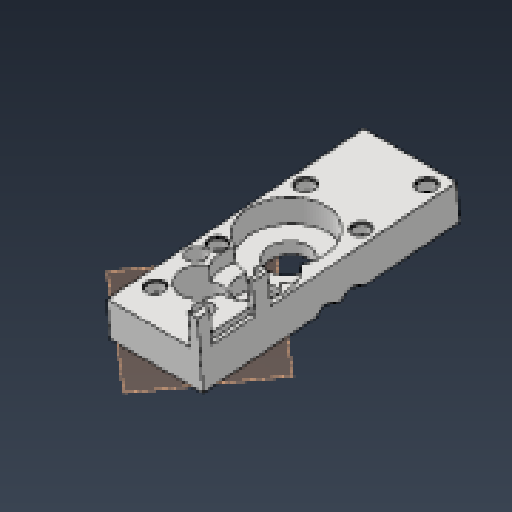
# Autodesk Inventor part: Right_gearbox
Saved by Autodesk Inventor 2026.2 (Build 302298010, 298A)
## iProperties
Created: 2026-04-04
Part Number: Right_gearbox
Material: Generic
Document SubType Name: Modeling
Designer: szymo
Density: 1 g/cm^3
Appearance: Default
Mass: 7.93657 g
Surface Area: 65.2995 cm^2
Volume: 7.93657 cm^3
Author: szymo
Autodesk Inventor part; units mm, degrees
(part 1 of 2)
ref_plane "YZ Plane" through (0, 0, 0) normal (1, 0, 0) x (0, 1, 0)
ref_plane "XZ Plane" through (0, 0, 0) normal (0, 1, 0) x (-1, 0, 0)
ref_plane "XY Plane" through (0, 0, 0) normal (0, 0, 1) x (1, 0, 0)
ref_plane "Work Plane1" through (-23.7091, -17.2437, 13.99) normal (0, 0.9970894, 0.0762418) x (-1, 0, 0)
sketch "Sketch1" plane through (-23.7091, -17.2437, 13.99) normal (0, 0.9970894, 0.0762418) x (-1, 0, 0)
  line L0 (-0.0409, -0.625) -> (23.5591, -0.625)
  line L1 (23.5591, -0.625) -> (23.5591, -65.9208)
  line L2 (23.5591, -65.9208) -> (-0.0409, -65.9208)
  line L3 (-0.0409, -65.9208) -> (-0.0409, -0.625)
  circle A0 centre (9.1675, -23.6102) radius 8 construction
  circle A1 centre (12.9591, -35.6262) radius 9.6 construction
  circle A2 centre (9.1675, -23.6102) radius 8.4
  circle A3 centre (12.9591, -35.6262) radius 10
  circle A4 centre (9.1675, -23.6102) radius 4.2 construction
  circle A5 centre (9.1675, -23.6102) radius 4.6
  line L4 (20.6624, -53.9792) -> (25.4482, -49.9634)
  arc A6 (25.4482, -49.9634) -> (22.2343, -46.1332) centre (14.4591, -55.9208) ccw
  line L5 (22.2343, -46.1332) -> (17.4484, -50.149)
  arc A7 (20.6624, -53.9792) -> (17.4484, -50.149) centre (14.4591, -55.9208) ccw
  arc A8 (3.4701, -61.8782) -> (6.684, -65.7084) centre (14.4591, -55.9208) ccw
  line L6 (3.4701, -61.8782) -> (8.2559, -57.8624)
  arc A9 (8.2559, -57.8624) -> (11.4698, -61.6927) centre (14.4591, -55.9208) ccw
  line L7 (11.4698, -61.6927) -> (6.684, -65.7084)
  line L8 (6.684, -65.7084) -> (6.684, -65.9208)
  line L9 (11.4698, -61.6927) -> (23.5591, -61.6927)
  circle A10 centre (14.4591, -15.125) radius 5 projected
  circle A11 centre (14.4591, -15.125) radius 13.85 construction
  circle A12 centre (14.4591, -55.9208) radius 14.5 construction
  circle A13 centre (14.4591, -15.125) radius 14.5 construction
  line L10 (19.1242, -50.0482) -> (22.2292, -47.4428) construction
  arc A14 (24.1576, -49.741) -> (22.2292, -47.4428) centre (14.4591, -55.9208) ccw construction
  line L11 (24.1576, -49.741) -> (21.0526, -52.3464) construction
  arc A15 (21.0526, -52.3464) -> (19.1242, -50.0482) centre (14.4591, -55.9208) ccw construction
  arc A16 (4.7607, -62.1007) -> (6.6891, -64.3988) centre (14.4591, -55.9208) ccw construction
  line L12 (4.7607, -62.1007) -> (7.8657, -59.4953) construction
  arc A17 (7.8657, -59.4953) -> (9.7941, -61.7934) centre (14.4591, -55.9208) ccw construction
  line L13 (9.7941, -61.7934) -> (6.6891, -64.3988) construction
  circle A18 centre (14.4591, -55.9208) radius 5 projected
  circle A19 centre (14.4591, -55.9208) radius 13.85 projected
  circle A20 centre (12.9591, -35.6262) radius 5 projected
  circle A21 centre (9.1675, -23.6102) radius 1.25 projected
  arc A22 (5.3654, -25.3945) -> (6.7676, -25.1474) centre (5.4355, -21.6906) ccw projected
  arc A23 (6.7676, -25.1474) -> (6.9888, -25.4475) centre (9.1675, -23.6102) ccw projected
  arc A24 (6.9888, -25.4475) -> (6.3377, -26.7137) centre (9.8963, -27.7432) ccw projected
  arc A25 (6.3377, -26.7137) -> (6.767, -27.0565) centre (9.1675, -23.6102) ccw projected
  arc A26 (6.767, -27.0565) -> (7.8577, -26.1414) centre (4.9757, -23.8138) ccw projected
  arc A27 (7.8577, -26.1414) -> (8.1993, -26.2907) centre (9.1675, -23.6102) ccw projected
  arc A28 (8.1993, -26.2907) -> (8.2685, -27.7129) centre (11.8651, -26.8251) ccw projected
  arc A29 (8.2685, -27.7129) -> (8.8117, -27.7951) centre (9.1675, -23.6102) ccw projected
  arc A30 (8.8117, -27.7951) -> (9.2988, -26.4572) centre (5.6391, -25.8824) ccw projected
  arc A31 (9.2988, -26.4572) -> (9.6693, -26.4157) centre (9.1675, -23.6102) ccw projected
  arc A32 (9.6693, -26.4157) -> (10.4403, -27.6127) centre (13.1112, -25.0456) ccw projected
  arc A33 (10.4403, -27.6127) -> (10.9519, -27.4123) centre (9.1675, -23.6102) ccw projected
  arc A34 (10.9519, -27.4123) -> (10.7047, -26.0101) centre (7.248, -27.3422) ccw projected
  arc A35 (10.7047, -26.0101) -> (11.0048, -25.7889) centre (9.1675, -23.6102) ccw projected
  arc A36 (11.0048, -25.7889) -> (12.271, -26.4401) centre (13.3005, -22.8814) ccw projected
  arc A37 (12.271, -26.4401) -> (12.6139, -26.0108) centre (9.1675, -23.6102) ccw projected
  arc A38 (12.6139, -26.0108) -> (11.6987, -24.92) centre (9.3712, -27.802) ccw projected
  arc A39 (11.6987, -24.92) -> (11.848, -24.5784) centre (9.1675, -23.6102) ccw projected
  arc A40 (11.848, -24.5784) -> (13.2702, -24.5092) centre (12.3824, -20.9126) ccw projected
  arc A41 (13.2702, -24.5092) -> (13.3524, -23.966) centre (9.1675, -23.6102) ccw projected
  arc A42 (13.3524, -23.966) -> (12.0145, -23.4789) centre (11.4398, -27.1386) ccw projected
  arc A43 (12.0145, -23.4789) -> (11.973, -23.1084) centre (9.1675, -23.6102) ccw projected
  arc A44 (11.973, -23.1084) -> (13.17, -22.3374) centre (10.6029, -19.6665) ccw projected
  arc A45 (13.17, -22.3374) -> (12.9697, -21.8259) centre (9.1675, -23.6102) ccw projected
  arc A46 (12.9697, -21.8259) -> (11.5674, -22.073) centre (12.8996, -25.5298) ccw projected
  arc A47 (11.5674, -22.073) -> (11.3463, -21.7729) centre (9.1675, -23.6102) ccw projected
  arc A48 (11.3463, -21.7729) -> (11.9974, -20.5067) centre (8.4388, -19.4772) ccw projected
  arc A49 (11.9974, -20.5067) -> (11.5681, -20.1639) centre (9.1675, -23.6102) ccw projected
  arc A50 (11.5681, -20.1639) -> (10.4773, -21.079) centre (13.3593, -23.4066) ccw projected
  arc A51 (10.4773, -21.079) -> (10.1357, -20.9297) centre (9.1675, -23.6102) ccw projected
  arc A52 (10.1357, -20.9297) -> (10.0665, -19.5075) centre (6.4699, -20.3953) ccw projected
  arc A53 (10.0665, -19.5075) -> (9.5233, -19.4253) centre (9.1675, -23.6102) ccw projected
  arc A54 (9.5233, -19.4253) -> (9.0362, -20.7632) centre (12.6959, -21.3379) ccw projected
  arc A55 (9.0362, -20.7632) -> (8.6657, -20.8047) centre (9.1675, -23.6102) ccw projected
  arc A56 (8.6657, -20.8047) -> (7.8947, -19.6077) centre (5.2239, -22.1748) ccw projected
  arc A57 (7.8947, -19.6077) -> (7.3832, -19.8081) centre (9.1675, -23.6102) ccw projected
  arc A58 (7.3832, -19.8081) -> (7.6303, -21.2103) centre (11.0871, -19.8782) ccw projected
  arc A59 (7.6303, -21.2103) -> (7.3302, -21.4315) centre (9.1675, -23.6102) ccw projected
  arc A60 (7.3302, -21.4315) -> (6.064, -20.7803) centre (5.0345, -24.339) ccw projected
  arc A61 (6.064, -20.7803) -> (5.7212, -21.2096) centre (9.1675, -23.6102) ccw projected
  arc A62 (5.7212, -21.2096) -> (6.6363, -22.3004) centre (8.9639, -19.4184) ccw projected
  arc A63 (6.6363, -22.3004) -> (6.487, -22.642) centre (9.1675, -23.6102) ccw projected
  arc A64 (6.487, -22.642) -> (5.0649, -22.7112) centre (5.9526, -26.3078) ccw projected
  arc A65 (5.0649, -22.7112) -> (4.9826, -23.2544) centre (9.1675, -23.6102) ccw projected
  arc A66 (4.9826, -23.2544) -> (6.3206, -23.7415) centre (6.8953, -20.0818) ccw projected
  arc A67 (6.3206, -23.7415) -> (6.362, -24.112) centre (9.1675, -23.6102) ccw projected
  arc A68 (6.362, -24.112) -> (5.165, -24.883) centre (7.7322, -27.5539) ccw projected
  arc A69 (5.165, -24.883) -> (5.3654, -25.3945) centre (9.1675, -23.6102) ccw projected
  circle A70 centre (9.1675, -23.6102) radius 1.25 projected
  arc A71 (17.1384, -22.9282) -> (15.9774, -22.6664) centre (15.4653, -27.6426) ccw projected
  arc A72 (15.9774, -22.6664) -> (15.9187, -22.3113) centre (9.1675, -23.6102) ccw projected
  arc A73 (15.9187, -22.3113) -> (16.9336, -21.6897) centre (13.8318, -17.7649) ccw projected
  arc A74 (16.9336, -21.6897) -> (16.8224, -21.2858) centre (9.1675, -23.6102) ccw projected
  arc A75 (16.8224, -21.2858) -> (15.6324, -21.2712) centre (16.1661, -26.2451) ccw projected
  arc A76 (15.6324, -21.2712) -> (15.5011, -20.936) centre (9.1675, -23.6102) ccw projected
  arc A77 (15.5011, -20.936) -> (16.3646, -20.117) centre (12.5145, -16.9228) ccw projected
  arc A78 (16.3646, -20.117) -> (16.1719, -19.7451) centre (9.1675, -23.6102) ccw projected
  arc A79 (16.1719, -19.7451) -> (15.0048, -19.9781) centre (16.561, -24.7325) ccw projected
  arc A80 (15.0048, -19.9781) -> (14.8067, -19.6776) centre (9.1675, -23.6102) ccw projected
  arc A81 (14.8067, -19.6776) -> (15.481, -18.697) centre (11.051, -16.3731) ccw projected
  arc A82 (15.481, -18.697) -> (15.2152, -18.3733) centre (9.1675, -23.6102) ccw projected
  arc A83 (15.2152, -18.3733) -> (14.1221, -18.8439) centre (16.6328, -23.1708) ccw projected
  arc A84 (14.1221, -18.8439) -> (13.8659, -18.5911) centre (9.1675, -23.6102) ccw projected
  arc A85 (13.8659, -18.5911) -> (14.3215, -17.4917) centre (9.5052, -16.1397) ccw projected
  arc A86 (14.3215, -17.4917) -> (13.9942, -17.2303) centre (9.1675, -23.6102) ccw projected
  arc A87 (13.9942, -17.2303) -> (13.0229, -17.9179) centre (16.3783, -21.6283) ccw projected
  arc A88 (13.0229, -17.9179) -> (12.7197, -17.7239) centre (9.1675, -23.6102) ccw projected
  arc A89 (12.7197, -17.7239) -> (12.9368, -16.5538) centre (7.9446, -16.2327) ccw projected
  arc A90 (12.9368, -16.5538) -> (12.5623, -16.3662) centre (9.1675, -23.6102) ccw projected
  arc A91 (12.5623, -16.3662) -> (11.7551, -17.2407) centre (15.8086, -20.1724) ccw projected
  arc A92 (11.7551, -17.2407) -> (11.4182, -17.114) centre (9.1675, -23.6102) ccw projected
  arc A93 (11.4182, -17.114) -> (11.3873, -15.9243) centre (6.4374, -16.6482) ccw projected
  arc A94 (11.3873, -15.9243) -> (10.982, -15.8187) centre (9.1675, -23.6102) ccw projected
  arc A95 (10.982, -15.8187) -> (10.3743, -16.8419) centre (14.9487, -18.8667) ccw projected
  arc A96 (10.3743, -16.8419) -> (10.0184, -16.7881) centre (9.1675, -23.6102) ccw projected
  arc A97 (10.0184, -16.7881) -> (9.7408, -15.6308) centre (5.0496, -17.3679) ccw projected
  arc A98 (9.7408, -15.6308) -> (9.3224, -15.6117) centre (9.1675, -23.6102) ccw projected
  arc A99 (9.3224, -15.6117) -> (8.9407, -16.7389) centre (13.8362, -17.7684) ccw projected
  arc A100 (8.9407, -16.7389) -> (8.5814, -16.7602) centre (9.1675, -23.6102) ccw projected
  arc A101 (8.5814, -16.7602) -> (8.0693, -15.6859) centre (3.8418, -18.3605) ccw projected
  arc A102 (8.0693, -15.6859) -> (7.6561, -15.7543) centre (9.1675, -23.6102) ccw projected
  arc A103 (7.6561, -15.7543) -> (7.5171, -16.9362) centre (12.5196, -16.9254) ccw projected
  arc A104 (7.5171, -16.9362) -> (7.17, -17.0318) centre (9.1675, -23.6102) ccw projected
  arc A105 (7.17, -17.0318) -> (6.4457, -16.0874) centre (2.8667, -19.5825) ccw projected
  arc A106 (6.4457, -16.0874) -> (6.0558, -16.2402) centre (9.1675, -23.6102) ccw projected
  arc A107 (6.0558, -16.2402) -> (6.1655, -17.4252) centre (11.0565, -16.3745) ccw projected
  arc A108 (6.1655, -17.4252) -> (5.846, -17.5908) centre (9.1675, -23.6102) ccw projected
  arc A109 (5.846, -17.5908) -> (4.9411, -16.8177) centre (2.167, -20.9806) ccw projected
  arc A110 (4.9411, -16.8177) -> (4.5914, -17.0482) centre (9.1675, -23.6102) ccw projected
  arc A111 (4.5914, -17.0482) -> (4.9452, -18.1845) centre (9.5108, -16.1399) ccw projected
  arc A112 (4.9452, -18.1845) -> (4.667, -18.413) centre (9.1675, -23.6102) ccw projected
  arc A113 (4.667, -18.413) -> (3.6213, -17.8449) centre (1.7732, -22.4935) ccw projected
  arc A114 (3.6213, -17.8449) -> (3.3271, -18.143) centre (9.1675, -23.6102) ccw projected
  arc A115 (3.3271, -18.143) -> (3.9094, -19.181) centre (7.9502, -16.2318) ccw projected
  arc A116 (3.9094, -19.181) -> (3.6848, -19.4622) centre (9.1675, -23.6102) ccw projected
  arc A117 (3.6848, -19.4622) -> (2.5438, -19.124) centre (1.7026, -24.0553) ccw projected
  arc A118 (2.5438, -19.124) -> (2.3181, -19.4768) centre (9.1675, -23.6102) ccw projected
  arc A119 (2.3181, -19.4768) -> (3.1034, -20.371) centre (6.4427, -16.6461) ccw projected
  arc A120 (3.1034, -20.371) -> (2.9422, -20.6928) centre (9.1675, -23.6102) ccw projected
  arc A121 (2.9422, -20.6928) -> (1.7558, -20.5992) centre (1.9583, -25.5976) ccw projected
  arc A122 (1.7558, -20.5992) -> (1.6084, -20.9912) centre (9.1675, -23.6102) ccw projected
  arc A123 (1.6084, -20.9912) -> (2.5625, -21.7026) centre (5.0543, -17.3648) ccw projected
  arc A124 (2.5625, -21.7026) -> (2.4717, -22.0509) centre (9.1675, -23.6102) ccw projected
  arc A125 (2.4717, -22.0509) -> (1.2917, -22.206) centre (2.529, -27.0531) ccw projected
  arc A126 (1.2917, -22.206) -> (1.229, -22.6201) centre (9.1675, -23.6102) ccw projected
  arc A127 (1.229, -22.6201) -> (2.3102, -23.1175) centre (3.8457, -18.3565) ccw projected
  arc A128 (2.3102, -23.1175) -> (2.2938, -23.4771) centre (9.1675, -23.6102) ccw projected
  arc A129 (2.2938, -23.4771) -> (1.1719, -23.8741) centre (3.3899, -28.3581) ccw projected
  arc A130 (1.1719, -23.8741) -> (1.1967, -24.2922) centre (9.1675, -23.6102) ccw projected
  arc A131 (1.1967, -24.2922) -> (2.3576, -24.554) centre (2.8697, -19.5777) ccw projected
  arc A132 (2.3576, -24.554) -> (2.4163, -24.9091) centre (9.1675, -23.6102) ccw projected
  arc A133 (2.4163, -24.9091) -> (1.4015, -25.5307) centre (4.5033, -29.4555) ccw projected
  arc A134 (1.4015, -25.5307) -> (1.5126, -25.9345) centre (9.1675, -23.6102) ccw projected
  arc A135 (1.5126, -25.9345) -> (2.7027, -25.9492) centre (2.169, -20.9752) ccw projected
  arc A136 (2.7027, -25.9492) -> (2.8339, -26.2844) centre (9.1675, -23.6102) ccw projected
  arc A137 (2.8339, -26.2844) -> (1.9705, -27.1034) centre (5.8205, -30.2975) ccw projected
  arc A138 (1.9705, -27.1034) -> (2.1632, -27.4753) centre (9.1675, -23.6102) ccw projected
  arc A139 (2.1632, -27.4753) -> (3.3302, -27.2422) centre (1.7741, -22.4879) ccw projected
  arc A140 (3.3302, -27.2422) -> (3.5283, -27.5428) centre (9.1675, -23.6102) ccw projected
  arc A141 (3.5283, -27.5428) -> (2.854, -28.5234) centre (7.2841, -30.8473) ccw projected
  arc A142 (2.854, -28.5234) -> (3.1198, -28.8471) centre (9.1675, -23.6102) ccw projected
  arc A143 (3.1198, -28.8471) -> (4.213, -28.3765) centre (1.7023, -24.0496) ccw projected
  arc A144 (4.213, -28.3765) -> (4.4692, -28.6293) centre (9.1675, -23.6102) ccw projected
  arc A145 (4.4692, -28.6293) -> (4.0135, -29.7287) centre (8.8299, -31.0807) ccw projected
  arc A146 (4.0135, -29.7287) -> (4.3408, -29.9901) centre (9.1675, -23.6102) ccw projected
  arc A147 (4.3408, -29.9901) -> (5.3122, -29.3025) centre (1.9568, -25.5921) ccw projected
  arc A148 (5.3122, -29.3025) -> (5.6154, -29.4964) centre (9.1675, -23.6102) ccw projected
  arc A149 (5.6154, -29.4964) -> (5.3983, -30.6666) centre (10.3905, -30.9877) ccw projected
  arc A150 (5.3983, -30.6666) -> (5.7727, -30.8542) centre (9.1675, -23.6102) ccw projected
  arc A151 (5.7727, -30.8542) -> (6.5799, -29.9797) centre (2.5264, -27.048) ccw projected
  arc A152 (6.5799, -29.9797) -> (6.9168, -30.1063) centre (9.1675, -23.6102) ccw projected
  arc A153 (6.9168, -30.1063) -> (6.9477, -31.2961) centre (11.8976, -30.5722) ccw projected
  arc A154 (6.9477, -31.2961) -> (7.353, -31.4017) centre (9.1675, -23.6102) ccw projected
  arc A155 (7.353, -31.4017) -> (7.9608, -30.3785) centre (3.3863, -28.3537) ccw projected
  arc A156 (7.9608, -30.3785) -> (8.3166, -30.4323) centre (9.1675, -23.6102) ccw projected
  arc A157 (8.3166, -30.4323) -> (8.5942, -31.5896) centre (13.2855, -29.8524) ccw projected
  arc A158 (8.5942, -31.5896) -> (9.0126, -31.6087) centre (9.1675, -23.6102) ccw projected
  arc A159 (9.0126, -31.6087) -> (9.3943, -30.4815) centre (4.4989, -29.452) ccw projected
  arc A160 (9.3943, -30.4815) -> (9.7536, -30.4602) centre (9.1675, -23.6102) ccw projected
  arc A161 (9.7536, -30.4602) -> (10.2658, -31.5345) centre (14.4933, -28.8599) ccw projected
  arc A162 (10.2658, -31.5345) -> (10.679, -31.4661) centre (9.1675, -23.6102) ccw projected
  arc A163 (10.679, -31.4661) -> (10.818, -30.2841) centre (5.8155, -30.295) ccw projected
  arc A164 (10.818, -30.2841) -> (11.165, -30.1886) centre (9.1675, -23.6102) ccw projected
  arc A165 (11.165, -30.1886) -> (11.8893, -31.1329) centre (15.4684, -27.6379) ccw projected
  arc A166 (11.8893, -31.1329) -> (12.2793, -30.9802) centre (9.1675, -23.6102) ccw projected
  arc A167 (12.2793, -30.9802) -> (12.1695, -29.7952) centre (7.2786, -30.8459) ccw projected
  arc A168 (12.1695, -29.7952) -> (12.4891, -29.6296) centre (9.1675, -23.6102) ccw projected
  arc A169 (12.4891, -29.6296) -> (13.3939, -30.4027) centre (16.1681, -26.2398) ccw projected
  arc A170 (13.3939, -30.4027) -> (13.7436, -30.1722) centre (9.1675, -23.6102) ccw projected
  arc A171 (13.7436, -30.1722) -> (13.3898, -29.0358) centre (8.8242, -31.0805) ccw projected
  arc A172 (13.3898, -29.0358) -> (13.668, -28.8074) centre (9.1675, -23.6102) ccw projected
  arc A173 (13.668, -28.8074) -> (14.7138, -29.3755) centre (16.5619, -24.7269) ccw projected
  arc A174 (14.7138, -29.3755) -> (15.0079, -29.0774) centre (9.1675, -23.6102) ccw projected
  arc A175 (15.0079, -29.0774) -> (14.4256, -28.0394) centre (10.3849, -30.9886) ccw projected
  arc A176 (14.4256, -28.0394) -> (14.6502, -27.7582) centre (9.1675, -23.6102) ccw projected
  arc A177 (14.6502, -27.7582) -> (15.7913, -28.0964) centre (16.6324, -23.1651) ccw projected
  arc A178 (15.7913, -28.0964) -> (16.017, -27.7436) centre (9.1675, -23.6102) ccw projected
  arc A179 (16.017, -27.7436) -> (15.2316, -26.8494) centre (11.8923, -30.5743) ccw projected
  arc A180 (15.2316, -26.8494) -> (15.3928, -26.5276) centre (9.1675, -23.6102) ccw projected
  arc A181 (15.3928, -26.5276) -> (16.5793, -26.6212) centre (16.3768, -21.6228) ccw projected
  arc A182 (16.5793, -26.6212) -> (16.7267, -26.2292) centre (9.1675, -23.6102) ccw projected
  arc A183 (16.7267, -26.2292) -> (15.7726, -25.5178) centre (13.2807, -29.8556) ccw projected
  arc A184 (15.7726, -25.5178) -> (15.8634, -25.1695) centre (9.1675, -23.6102) ccw projected
  arc A185 (15.8634, -25.1695) -> (17.0433, -25.0144) centre (15.806, -20.1673) ccw projected
  arc A186 (17.0433, -25.0144) -> (17.106, -24.6003) centre (9.1675, -23.6102) ccw projected
  arc A187 (17.106, -24.6003) -> (16.0249, -24.1029) centre (14.4893, -28.8639) ccw projected
  arc A188 (16.0249, -24.1029) -> (16.0412, -23.7433) centre (9.1675, -23.6102) ccw projected
  arc A189 (16.0412, -23.7433) -> (17.1632, -23.3463) centre (14.9451, -18.8623) ccw projected
  arc A190 (17.1632, -23.3463) -> (17.1384, -22.9282) centre (9.1675, -23.6102) ccw projected
  arc A191 (20.5914, -38.7585) -> (22.0189, -38.8013) centre (21.4836, -32.8221) ccw projected
  arc A192 (20.417, -39.1536) -> (20.5914, -38.7585) centre (12.9591, -35.6262) ccw projected
  arc A193 (21.4106, -40.1794) -> (20.417, -39.1536) centre (16.6327, -43.8136) ccw projected
  arc A194 (21.1608, -40.6155) -> (21.4106, -40.1794) centre (12.9591, -35.6262) ccw projected
  arc A195 (19.7733, -40.2769) -> (21.1608, -40.6155) centre (21.8803, -34.6557) ccw projected
  arc A196 (19.5206, -40.6271) -> (19.7733, -40.2769) centre (12.9591, -35.6262) ccw projected
  arc A197 (20.2793, -41.8371) -> (19.5206, -40.6271) centre (14.8501, -44.3985) ccw projected
  arc A198 (19.9442, -42.2117) -> (20.2793, -41.8371) centre (12.9591, -35.6262) ccw projected
  arc A199 (18.6575, -41.592) -> (19.9442, -42.2117) centre (21.8871, -36.5318) ccw projected
  arc A200 (18.3375, -41.8821) -> (18.6575, -41.592) centre (12.9591, -35.6262) ccw projected
  arc A201 (18.828, -43.2233) -> (18.3375, -41.8821) centre (12.9849, -44.5999) ccw projected
  arc A202 (18.4223, -43.52) -> (18.828, -43.2233) centre (12.9591, -35.6262) ccw projected
  arc A203 (17.2926, -42.6464) -> (18.4223, -43.52) centre (21.5037, -38.3682) ccw projected
  arc A204 (16.9193, -42.8636) -> (17.2926, -42.6464) centre (12.9591, -35.6262) ccw projected
  arc A205 (17.1202, -44.2775) -> (16.9193, -42.8636) centre (11.1186, -44.4092) ccw projected
  arc A206 (16.6617, -44.4834) -> (17.1202, -44.2775) centre (12.9591, -35.6262) ccw projected
  arc A207 (15.7383, -43.394) -> (16.6617, -44.4834) centre (20.7469, -40.0848) ccw projected
  arc A208 (15.328, -43.5288) -> (15.7383, -43.394) centre (12.9591, -35.6262) ccw projected
  arc A209 (15.2306, -44.9536) -> (15.328, -43.5288) centre (9.3327, -43.8346) ccw projected
  arc A210 (14.7393, -45.0597) -> (15.2306, -44.9536) centre (12.9591, -35.6262) ccw projected
  arc A211 (14.0626, -43.802) -> (14.7393, -45.0597) centre (19.6497, -41.6065) ccw projected
  arc A212 (13.6332, -43.8486) -> (14.0626, -43.802) centre (12.9591, -35.6262) ccw projected
  arc A213 (13.2417, -45.222) -> (13.6332, -43.8486) centre (7.7054, -42.9013) ccw projected
  arc A214 (12.7391, -45.2237) -> (13.2417, -45.222) centre (12.9591, -35.6262) ccw projected
  arc A215 (12.3386, -43.8528) -> (12.7391, -45.2237) centre (18.2601, -42.8669) ccw projected
  arc A216 (11.9089, -43.8091) -> (12.3386, -43.8528) centre (12.9591, -35.6262) ccw projected
  arc A217 (11.2404, -45.0711) -> (11.9089, -43.8091) centre (6.3076, -41.65) ccw projected
  arc A218 (10.7484, -44.9682) -> (11.2404, -45.0711) centre (12.9591, -35.6262) ccw projected
  arc A219 (10.6418, -43.544) -> (10.7484, -44.9682) centre (16.6389, -43.8108) ccw projected
  arc A220 (10.2305, -43.4119) -> (10.6418, -43.544) centre (12.9591, -35.6262) ccw projected
  arc A221 (9.3143, -44.5073) -> (10.2305, -43.4119) centre (5.2005, -40.1354) ccw projected
  arc A222 (8.8544, -44.3044) -> (9.3143, -44.5073) centre (12.9591, -35.6262) ccw projected
  arc A223 (9.0462, -42.8892) -> (8.8544, -44.3044) centre (14.8568, -44.397) ccw projected
  arc A224 (8.6714, -42.6744) -> (9.0462, -42.8892) centre (12.9591, -35.6262) ccw projected
  arc A225 (7.5474, -43.5554) -> (8.6714, -42.6744) centre (4.4325, -38.4238) ccw projected
  arc A226 (7.1398, -43.2613) -> (7.5474, -43.5554) centre (12.9591, -35.6262) ccw projected
  arc A227 (7.6216, -41.9169) -> (7.1398, -43.2613) centre (12.9917, -44.5999) ccw projected
  arc A228 (7.2997, -41.629) -> (7.6216, -41.9169) centre (12.9591, -35.6262) ccw projected
  arc A229 (6.0171, -42.257) -> (7.2997, -41.629) centre (4.0372, -36.5898) ccw projected
  arc A230 (5.6796, -41.8846) -> (6.0171, -42.257) centre (12.9591, -35.6262) ccw projected
  arc A231 (6.4303, -40.6697) -> (5.6796, -41.8846) centre (11.1253, -44.4106) ccw projected
  arc A232 (6.1753, -40.3211) -> (6.4303, -40.6697) centre (12.9591, -35.6262) ccw projected
  arc A233 (4.7902, -40.6688) -> (6.1753, -40.3211) centre (4.0318, -34.7138) ccw projected
  arc A234 (4.5374, -40.2343) -> (4.7902, -40.6688) centre (12.9591, -35.6262) ccw projected
  arc A235 (5.5244, -39.2021) -> (4.5374, -40.2343) centre (9.339, -43.8374) ccw projected
  arc A236 (5.3474, -38.8081) -> (5.5244, -39.2021) centre (12.9591, -35.6262) ccw projected
  arc A237 (3.9202, -38.8602) -> (5.3474, -38.8081) centre (4.4166, -32.8777) ccw projected
  arc A238 (3.7634, -38.3827) -> (3.9202, -38.8602) centre (12.9591, -35.6262) ccw projected
  arc A239 (4.9434, -37.5782) -> (3.7634, -38.3827) centre (7.7109, -42.9053) ccw projected
  arc A240 (4.8522, -37.156) -> (4.9434, -37.5782) centre (12.9591, -35.6262) ccw projected
  arc A241 (3.4454, -36.9102) -> (4.8522, -37.156) centre (5.1747, -31.1616) ccw projected
  arc A242 (3.3912, -36.4105) -> (3.4454, -36.9102) centre (12.9591, -35.6262) ccw projected
  arc A243 (4.7127, -35.869) -> (3.3912, -36.4105) centre (6.3122, -41.655) ccw projected
  arc A244 (4.7113, -35.4371) -> (4.7127, -35.869) centre (12.9591, -35.6262) ccw projected
  arc A245 (3.3863, -34.9041) -> (4.7113, -35.4371) centre (6.2731, -29.6407) ccw projected
  arc A246 (3.4372, -34.4041) -> (3.3863, -34.9041) centre (12.9591, -35.6262) ccw projected
  arc A247 (4.8424, -34.1491) -> (3.4372, -34.4041) centre (5.2039, -40.1413) ccw projected
  arc A248 (4.9309, -33.7264) -> (4.8424, -34.1491) centre (12.9591, -35.6262) ccw projected
  arc A249 (3.7456, -32.9296) -> (4.9309, -33.7264) centre (7.6636, -28.3814) ccw projected
  arc A250 (3.8994, -32.4511) -> (3.7456, -32.9296) centre (12.9591, -35.6262) ccw projected
  arc A251 (5.3269, -32.4939) -> (3.8994, -32.4511) centre (4.4347, -38.4302) ccw projected
  arc A252 (5.5013, -32.0987) -> (5.3269, -32.4939) centre (12.9591, -35.6262) ccw projected
  arc A253 (4.5076, -31.0729) -> (5.5013, -32.0987) centre (9.2856, -27.4387) ccw projected
  arc A254 (4.7575, -30.6369) -> (4.5076, -31.0729) centre (12.9591, -35.6262) ccw projected
  arc A255 (6.1449, -30.9755) -> (4.7575, -30.6369) centre (4.038, -36.5966) ccw projected
  arc A256 (6.3977, -30.6252) -> (6.1449, -30.9755) centre (12.9591, -35.6262) ccw projected
  arc A257 (5.639, -29.4153) -> (6.3977, -30.6252) centre (11.0681, -26.8539) ccw projected
  arc A258 (5.9741, -29.0407) -> (5.639, -29.4153) centre (12.9591, -35.6262) ccw projected
  arc A259 (7.2608, -29.6603) -> (5.9741, -29.0407) centre (4.0311, -34.7206) ccw projected
  arc A260 (7.5808, -29.3703) -> (7.2608, -29.6603) centre (12.9591, -35.6262) ccw projected
  arc A261 (7.0903, -28.029) -> (7.5808, -29.3703) centre (12.9333, -26.6524) ccw projected
  arc A262 (7.4959, -27.7323) -> (7.0903, -28.029) centre (12.9591, -35.6262) ccw projected
  arc A263 (8.6256, -28.606) -> (7.4959, -27.7323) centre (4.4145, -32.8842) ccw projected
  arc A264 (8.999, -28.3888) -> (8.6256, -28.606) centre (12.9591, -35.6262) ccw projected
  arc A265 (8.798, -26.9749) -> (8.999, -28.3888) centre (14.7996, -26.8431) ccw projected
  arc A266 (9.2565, -26.7689) -> (8.798, -26.9749) centre (12.9591, -35.6262) ccw projected
  arc A267 (10.1799, -27.8584) -> (9.2565, -26.7689) centre (5.1713, -31.1675) ccw projected
  arc A268 (10.5903, -27.7236) -> (10.1799, -27.8584) centre (12.9591, -35.6262) ccw projected
  arc A269 (10.6877, -26.2988) -> (10.5903, -27.7236) centre (16.5855, -27.4177) ccw projected
  arc A270 (11.179, -26.1927) -> (10.6877, -26.2988) centre (12.9591, -35.6262) ccw projected
  arc A271 (11.8557, -27.4503) -> (11.179, -26.1927) centre (6.2685, -29.6458) ccw projected
  arc A272 (12.2851, -27.4038) -> (11.8557, -27.4503) centre (12.9591, -35.6262) ccw projected
  arc A273 (12.6766, -26.0303) -> (12.2851, -27.4038) centre (18.2129, -28.3511) ccw projected
  arc A274 (13.1792, -26.0287) -> (12.6766, -26.0303) centre (12.9591, -35.6262) ccw projected
  arc A275 (13.5796, -27.3995) -> (13.1792, -26.0287) centre (7.6581, -28.3854) ccw projected
  arc A276 (14.0093, -27.4433) -> (13.5796, -27.3995) centre (12.9591, -35.6262) ccw projected
  arc A277 (14.6779, -26.1813) -> (14.0093, -27.4433) centre (19.6107, -29.6024) ccw projected
  arc A278 (15.1698, -26.2842) -> (14.6779, -26.1813) centre (12.9591, -35.6262) ccw projected
  arc A279 (15.2765, -27.7083) -> (15.1698, -26.2842) centre (9.2794, -27.4415) ccw projected
  arc A280 (15.6877, -27.8405) -> (15.2765, -27.7083) centre (12.9591, -35.6262) ccw projected
  arc A281 (16.604, -26.745) -> (15.6877, -27.8405) centre (20.7177, -31.117) ccw projected
  arc A282 (17.0638, -26.948) -> (16.604, -26.745) centre (12.9591, -35.6262) ccw projected
  arc A283 (16.8721, -28.3632) -> (17.0638, -26.948) centre (11.0615, -26.8553) ccw projected
  arc A284 (17.2468, -28.5779) -> (16.8721, -28.3632) centre (12.9591, -35.6262) ccw projected
  arc A285 (18.3709, -27.6969) -> (17.2468, -28.5779) centre (21.4857, -32.8286) ccw projected
  arc A286 (18.7784, -27.991) -> (18.3709, -27.6969) centre (12.9591, -35.6262) ccw projected
  arc A287 (18.2966, -29.3354) -> (18.7784, -27.991) centre (12.9265, -26.6524) ccw projected
  arc A288 (18.6186, -29.6234) -> (18.2966, -29.3354) centre (12.9591, -35.6262) ccw projected
  arc A289 (19.9012, -28.9953) -> (18.6186, -29.6234) centre (21.881, -34.6625) ccw projected
  arc A290 (20.2387, -29.3677) -> (19.9012, -28.9953) centre (12.9591, -35.6262) ccw projected
  arc A291 (19.4879, -30.5826) -> (20.2387, -29.3677) centre (14.793, -26.8417) ccw projected
  arc A292 (19.7429, -30.9312) -> (19.4879, -30.5826) centre (12.9591, -35.6262) ccw projected
  arc A293 (21.1281, -30.5836) -> (19.7429, -30.9312) centre (21.8864, -36.5385) ccw projected
  arc A294 (21.3808, -31.018) -> (21.1281, -30.5836) centre (12.9591, -35.6262) ccw projected
  arc A295 (20.3939, -32.0502) -> (21.3808, -31.018) centre (16.5793, -27.415) ccw projected
  arc A296 (20.5708, -32.4442) -> (20.3939, -32.0502) centre (12.9591, -35.6262) ccw projected
  arc A297 (21.998, -32.3922) -> (20.5708, -32.4442) centre (21.5017, -38.3747) ccw projected
  arc A298 (22.1549, -32.8697) -> (21.998, -32.3922) centre (12.9591, -35.6262) ccw projected
  arc A299 (20.9749, -33.6742) -> (22.1549, -32.8697) centre (18.2074, -28.3471) ccw projected
  arc A300 (21.066, -34.0963) -> (20.9749, -33.6742) centre (12.9591, -35.6262) ccw projected
  arc A301 (22.4729, -34.3422) -> (21.066, -34.0963) centre (20.7435, -40.0907) ccw projected
  arc A302 (22.527, -34.8418) -> (22.4729, -34.3422) centre (12.9591, -35.6262) ccw projected
  arc A303 (21.2056, -35.3834) -> (22.527, -34.8418) centre (19.6061, -29.5973) ccw projected
  arc A304 (21.207, -35.8153) -> (21.2056, -35.3834) centre (12.9591, -35.6262) ccw projected
  arc A305 (22.5319, -36.3482) -> (21.207, -35.8153) centre (19.6452, -41.6116) ccw projected
  arc A306 (22.481, -36.8482) -> (22.5319, -36.3482) centre (12.9591, -35.6262) ccw projected
  arc A307 (21.0758, -37.1032) -> (22.481, -36.8482) centre (20.7143, -31.1111) ccw projected
  arc A308 (20.9874, -37.526) -> (21.0758, -37.1032) centre (12.9591, -35.6262) ccw projected
  arc A309 (22.1726, -38.3228) -> (20.9874, -37.526) centre (18.2546, -42.8709) ccw projected
  arc A310 (22.0189, -38.8013) -> (22.1726, -38.3228) centre (12.9591, -35.6262) ccw projected
  point P0 (23.5591, -65.461)
  point P1 (4.3698, -30.5053)
  point P2 (17.0537, -26.5029)
  point P3 (13.2994, -25.632)
  point P4 (6.9443, -27.6373)
  point P5 (23.5591, -51.5485)
  point P6 (23.5591, -47.3511)
  point P7 (23.5591, -45.4799)
  point P8 (4.8767, -65.9208)
  point P9 (9.4599, -15.2153)
  point P10 (16.5776, -19.654)
  point P11 (19.6328, -43.0734)
  point P12 (7.4528, -43.9737)
  dimension "d0" = 0.4
  dimension "d1" = 0.4
  dimension "d3" = 0.6
  dimension "d108" = 0.4
  dimension "d131" = 1
  dimension "d132" = 1
  dimension "d133" = 1
  dimension "d134" = 1
  dimension "d135" = 1
  dimension "d136" = 1
  dimension "d137" = 1
  dimension "d138" = 1
  dimension "d139" = 4.5
  constraints: 20 end point, 9 point on circle, 8 centre point, 7 coincident, 3 perpendicular, 3 point on line, 2 parallel, 2 tangent, 1 horizontal, 6 other
  measures "d1" radial gap between concentric circles of A1 A3
  measures "d3" distance edge to line of A3 L1
  measures "d131" distance between parallel lines of L11 L4
  measures "d132" distance between parallel lines of L5 L10
  measures "d133" distance between parallel lines of L13 L7
  measures "d134" distance between parallel lines of L6 L12
  measures "d135" radial gap between concentric circles of A15 A7
  measures "d136" radial gap between concentric circles of A17 A9
  measures "d137" radial gap between concentric circles of A16 A8
  measures "d138" radial gap between concentric circles of A14 A6
  measures "d139" distance edge to line of A12 L2
ref_plane "Work Plane6" through (-57.5989, -15.4214, -20.1397) normal (0, 1, 0) x (-0.6427876, 0, 0.7660444)
ref_plane "Work Plane8" through (-57.5989, -16.7141, -20.4804) normal (0, 0.9970894, 0.0762418) x (-0.6427876, -0.0584046, 0.7638148)
extrude "Extrusion2" add sketch "Sketch1" against normal up to surface (2.1 mm away) contours L0 L1 A19 A3 A2 A10 L2 L3 | A19 A201 A200 A199 A198 A197 A196 A195 A194 A193 A192 A191 A310 A309 A308 A307 A306 A305 A304 A303 A302 A301 A300 A299 A298 A297 A296 A295 A294 A293 A292 A291 A290 A289 A288 A287 A286 A285 A284 A283 A282 A2 A3 | A3 A2 A254 A253 A252 A251 A250 A249 A248 A247 A246 A245 A244 A243 A242 A241 A240 A239 A238 A237 A236 A235 A234 A233 A232 A231 A230 A229 A228 A227 A226 A225 A224 A223 A19 | A19 A223 A224 A225 A226 A227 A228 A229 A230 A231 A232 A233 A234 A235 A236 A237 A238 A239 A240 A241 A242 A243 A244 A245 A246 A247 A248 A249 A250 A251 A252 A253 A254 A2 A20 A282 A283 A284 A285 A286 A287 A288 A289 A290 A291 A292 A293 A294 A295 A296 A297 A298 A299 A300 A301 A302 A303 A304 A305 A306 A307 A308 A309 A310 A191 A192 A193 A194 A195 A196 A197 A198 A199 A200 A201 | A3 A147 A148 A149 A150 A255 A254 A2 | A2 A10 A98 A99 A100 A101 A102 A103 A104 A105 A106 A107 A108 A109 A110 A111 A112 A113 A114 A115 A116 A117 A118 A119 A120 A121 A122 A123 A124 A125 A126 A127 A128 A129 A130 A131 A132 A133 A134 A135 A136 A137 A138 A139 A140 A141 A142 A143 A144 A145 A146 A147 A3 | A3 A182 A183 A184 A185 A186 A187 A188 A189 A190 A71 A72 A73 A74 A75 A76 A77 A78 A10 A2 | A2 A282 A281 A179 A279 A180 A181 A182 A3 | A254 A255 A150 A151 A256 A257 A152 A153 A154 A155 A156 A157 A158 A159 A160 A161 A20 A2 | A147 A146 A145 A144 A143 A142 A141 A140 A139 A138 A137 A136 A135 A134 A133 A132 A131 A130 A129 A128 A127 A126 A125 A124 A123 A122 A121 A120 A119 A118 A117 A116 A115 A114 A113 A112 A111 A110 A109 A108 A107 A106 A105 A104 A103 A102 A101 A100 A99 A98 A10 A78 A77 A76 A75 A74 A73 A72 A71 A190 A189 A188 A187 A186 A185 A184 A183 A182 A3 A5 | A3 A5 A262 A261 A260 A259 A258 A257 A151 A255 A150 A149 A148 A147 | A2 A20 A167 A168 A169 A170 A171 A172 A173 A174 A175 A176 A177 A178 A179 A281 A282 | A182 A181 A180 A279 A278 A277 A276 A275 A274 A5 A3 | A161 A160 A159 A158 A157 A156 A155 A154 A153 A152 A151 A257 A258 A259 A260 A261 A262 A5 A263 A264 A265 A271 A272 A273 A274 A275 A276 A277 A278 A279 A180 A179 A280 A281 A178 A177 A176 A175 A174 A173 A172 A171 A170 A169 A168 A167 A20 A165 A164 A163 | A255 A151 A150 | A281 A280 A279 A179 | A163 A164 A165 A20 | A151 A257 A256 A255 | A5 A265 A264 A263 | A179 A180 A279 | A273 A272 A271 A5
extrude "Extrusion3" add sketch "Sketch1" along normal blind 1 contours L0 L1 A19 A3 A2 A10 L2 L3 | A19 A201 A200 A199 A198 A197 A196 A195 A194 A193 A192 A191 A310 A309 A308 A307 A306 A305 A304 A303 A302 A301 A300 A299 A298 A297 A296 A295 A294 A293 A292 A291 A290 A289 A288 A287 A286 A285 A284 A283 A282 A2 A3 | A3 A19 A223 A222 A221 A220 A219 A218 A217 A216 A215 A214 A213 A212 A211 A210 A209 A208 A207 A206 A205 A204 A203 A202 A201 | A3 A2 A254 A253 A252 A251 A250 A249 A248 A247 A246 A245 A244 A243 A242 A241 A240 A239 A238 A237 A236 A235 A234 A233 A232 A231 A230 A229 A228 A227 A226 A225 A224 A223 A19 | A201 A202 A203 A204 A205 A206 A207 A208 A209 A210 A211 A212 A213 A214 A215 A216 A217 A218 A219 A220 A221 A222 A223 A19 | A19 A223 A224 A225 A226 A227 A228 A229 A230 A231 A232 A233 A234 A235 A236 A237 A238 A239 A240 A241 A242 A243 A244 A245 A246 A247 A248 A249 A250 A251 A252 A253 A254 A2 A20 A282 A283 A284 A285 A286 A287 A288 A289 A290 A291 A292 A293 A294 A295 A296 A297 A298 A299 A300 A301 A302 A303 A304 A305 A306 A307 A308 A309 A310 A191 A192 A193 A194 A195 A196 A197 A198 A199 A200 A201 | A3 A147 A148 A149 A150 A255 A254 A2 | A2 A10 A98 A99 A100 A101 A102 A103 A104 A105 A106 A107 A108 A109 A110 A111 A112 A113 A114 A115 A116 A117 A118 A119 A120 A121 A122 A123 A124 A125 A126 A127 A128 A129 A130 A131 A132 A133 A134 A135 A136 A137 A138 A139 A140 A141 A142 A143 A144 A145 A146 A147 A3 | A3 A182 A183 A184 A185 A186 A187 A188 A189 A190 A71 A72 A73 A74 A75 A76 A77 A78 A10 A2 | A2 A282 A281 A179 A279 A180 A181 A182 A3 | A254 A255 A150 A151 A256 A257 A152 A153 A154 A155 A156 A157 A158 A159 A160 A161 A20 A2 | A147 A146 A145 A144 A143 A142 A141 A140 A139 A138 A137 A136 A135 A134 A133 A132 A131 A130 A129 A128 A127 A126 A125 A124 A123 A122 A121 A120 A119 A118 A117 A116 A115 A114 A113 A112 A111 A110 A109 A108 A107 A106 A105 A104 A103 A102 A101 A100 A99 A98 A10 A78 A77 A76 A75 A74 A73 A72 A71 A190 A189 A188 A187 A186 A185 A184 A183 A182 A3 A5 | A3 A5 A262 A261 A260 A259 A258 A257 A151 A255 A150 A149 A148 A147 | A2 A20 A167 A168 A169 A170 A171 A172 A173 A174 A175 A176 A177 A178 A179 A281 A282 | A182 A181 A180 A279 A278 A277 A276 A275 A274 A5 A3 | A161 A160 A159 A158 A157 A156 A155 A154 A153 A152 A151 A257 A258 A259 A260 A261 A262 A5 A263 A264 A265 A271 A272 A273 A274 A275 A276 A277 A278 A279 A180 A179 A280 A281 A178 A177 A176 A175 A174 A173 A172 A171 A170 A169 A168 A167 A20 A165 A164 A163 | A255 A151 A150 | A281 A280 A279 A179 | A163 A164 A165 A20 | A151 A257 A256 A255 | A5 A265 A264 A263 | A179 A180 A279 | A273 A272 A271 A5
extrude "Extrusion4" add sketch "Sketch1" along normal blind 3.4 contours L0 L1 A19 A3 A2 A10 L2 L3 | L1 A6 L5 A7 L4 L9 A9 L6 A8 L8 L2 A19 A3 | A2 A10 A98 A99 A100 A101 A102 A103 A104 A105 A106 A107 A108 A109 A110 A111 A112 A113 A114 A115 A116 A117 A118 A119 A120 A121 A122 A123 A124 A125 A126 A127 A128 A129 A130 A131 A132 A133 A134 A135 A136 A137 A138 A139 A140 A141 A142 A143 A144 A145 A146 A147 A3 | A3 A182 A183 A184 A185 A186 A187 A188 A189 A190 A71 A72 A73 A74 A75 A76 A77 A78 A10 A2 | A147 A146 A145 A144 A143 A142 A141 A140 A139 A138 A137 A136 A135 A134 A133 A132 A131 A130 A129 A128 A127 A126 A125 A124 A123 A122 A121 A120 A119 A118 A117 A116 A115 A114 A113 A112 A111 A110 A109 A108 A107 A106 A105 A104 A103 A102 A101 A100 A99 A98 A10 A78 A77 A76 A75 A74 A73 A72 A71 A190 A189 A188 A187 A186 A185 A184 A183 A182 A3 A5